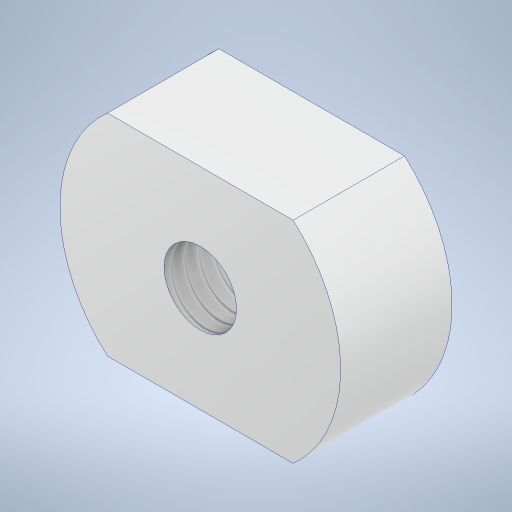
# Autodesk Inventor part: Print Bed Washers
Saved by Autodesk Inventor 2024 (Build 280153000, 153)
## iProperties
Created: 2024-08-03
Part Number: Print Bed Washers
Material: Aluminum 6061
Document SubType Name: Modeling
Designer: Ishaan
Density: 2.7 g/cm^3
Appearance: Aluminum - Flat
Author: Ishaan
Autodesk Inventor part; units mm, degrees
ref_plane "YZ Plane" through (0, 0, 0) normal (1, 0, 0) x (0, 1, 0)
ref_plane "XZ Plane" through (0, 0, 0) normal (0, 1, 0) x (-1, 0, 0)
ref_plane "XY Plane" through (0, 0, 0) normal (0, 0, 1) x (1, 0, 0)
sketch "Sketch1" plane through (0, 0, 0) normal (0, 0, 1) x (1, 0, 0)
  circle A0 centre (0, 0) radius 8
  line L0 (5.2915, -6) -> (-5.2915, -6)
  line L1 (-5.2915, -6) -> (-5.2915, 6)
  line L2 (-5.2915, 6) -> (5.2915, 6)
  line L3 (5.2915, 6) -> (5.2915, -6)
  line L4 (5.2915, -6) -> (-5.2915, 6) construction
  line L5 (-5.2915, -6) -> (5.2915, 6) construction
  point P0 (-5.2915, -6)
  point P1 (5.2915, -6)
  point P2 (5.2915, 6)
  dimension "d0" = 16
  dimension "d1" = 12
  constraints: 12 end point, 2 midpoint, 2 parallel, 1 coincident, 1 horizontal, 1 perpendicular, 3 other
  measures "d1" distance of L0.end L1.end
extrude "Extrusion1" add sketch "Sketch1" along normal blind 6.35 contours A0 L3 | L3 L0 L1 L2 | L1 A0
sketch "Sketch2" plane through (0, 0, 6.35) normal (0, 0, 1) x (1, 0, 0)
  arc A0 (-5.2915, 6) -> (-5.2915, -6) centre (0, 0) ccw projected
  constraints: 1 coincident
hole "Hole1" at (0, 0, 6.35) direction (0, 0, -1) diameter 4.134 end through all thread size "M5x0.8" class "6H" standard "ANSI Metric M Profile"
body "Solid1"
